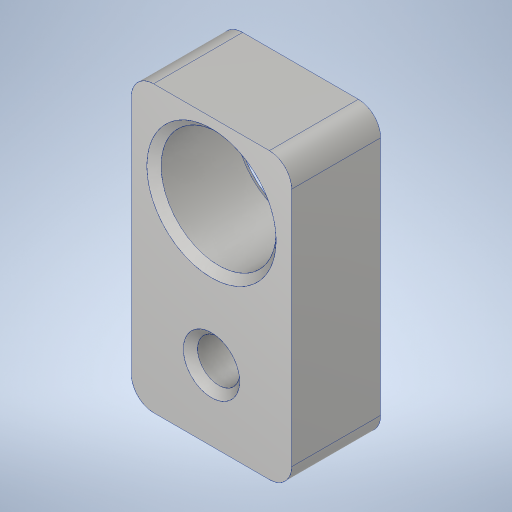
# Autodesk Inventor part: beam_break_spacer
Saved by Autodesk Inventor 2023.3 (Build 273359000, 359)
## iProperties
Created: 2024-02-24
Part Number: beam_break_spacer
Material: Aluminum 6061
Document SubType Name: Modeling
Designer: mavericks
Density: 2.7 g/cm^3
Appearance: Aluminum - Flat
Author: mavericks
Autodesk Inventor part; units mm, degrees
ref_plane "YZ Plane" through (0, 0, 0) normal (1, 0, 0) x (0, 1, 0)
ref_plane "XZ Plane" through (0, 0, 0) normal (0, 1, 0) x (-1, 0, 0)
ref_plane "XY Plane" through (0, 0, 0) normal (0, 0, 1) x (1, 0, 0)
sketch "Sketch1" plane through (0, 0, 0) normal (0, 0, 1) x (1, 0, 0)
  line L0 (-5.715, -10.16) -> (5.715, -10.16)
  line L1 (5.715, -10.16) -> (5.715, 10.16)
  line L2 (5.715, 10.16) -> (-5.715, 10.16)
  line L3 (-5.715, 10.16) -> (-5.715, -10.16)
  line L4 (-5.715, -10.16) -> (5.715, 10.16) construction
  line L5 (5.715, -10.16) -> (-5.715, 10.16) construction
  point P0 (0, 0)
  dimension "d0" = 20.32
  dimension "d1" = 11.43
  constraints: 12 end point, 2 midpoint, 2 parallel, 1 horizontal, 1 perpendicular
  measures "d0" distance of L2.end L0.start
  measures "d1" distance of L1.end L2.end
extrude "Extrusion1" add sketch "Sketch1" along normal blind 6.35
sketch "Sketch2" plane through (0, 0, 6.35) normal (0, 0, 1) x (1, 0, 0)
  line L0 (-5.715, 10.16) -> (-5.715, -10.16) projected
  line L1 (-5.715, -10.16) -> (5.715, -10.16) projected
  point P0 (0, 0)
  point P1 (0, -5.1562)
  dimension "d5" = 5.0038
  dimension "d22" = 5.715
  measures "d5" distance from line of L1 point (0, -5.156)
  measures "d22" distance from line of L0 point (0, -5.156)
hole "Hole1" at (0, -5.1562, 6.35) direction (0, 0, -1) diameter 3 end through all
sketch "Sketch3" plane through (0, 0, 6.35) normal (0, 0, 1) x (1, 0, 0)
  line L0 (-5.715, -10.16) -> (5.715, -10.16) projected
  line L1 (5.715, -10.16) -> (5.715, 10.16) projected
  point P0 (0, 0)
  point P1 (0, 4.848)
  dimension "d13" = 15.008
  dimension "d14" = 5.715
  measures "d13" distance from line of L0 point (0, 4.848)
  measures "d14" distance from line of point (0, 4.848) L1
hole "Hole2" at (0, 4.848, 6.35) direction (0, 0, -1) diameter 8.2 end through all
fillet "Fillet1" radius 1.5875 4 edges at (5.715, 10.16, 3.175) (-5.715, 10.16, 3.175) (5.715, -10.16, 3.175) (-5.715, -10.16, 3.175)
chamfer "Chamfer1" distance 0.508 angle 45 4 edges at (0, -3.6562, 6.35) (0, 8.948, 6.35) (0, 8.948, 0) (0, -3.6562, 0)
body "Solid1"
